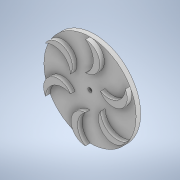
# Autodesk Inventor part: 20220608_ファン40mm羽数6枚
Saved by Autodesk Inventor 2020 (Build 240168000, 168)
## iProperties
Created: 2022-06-08
Part Number: 20220608_ファン40mm羽数6枚
Material: 一般
Document SubType Name: Modeling
Designer: Naggy
Density: 1 g/cm^3
Appearance: 既定
Author: Naggy
Autodesk Inventor part; units mm, degrees
ref_plane "YZ Plane" through (0, 0, 0) normal (1, 0, 0) x (0, 1, 0)
ref_plane "XZ Plane" through (0, 0, 0) normal (0, 1, 0) x (-1, 0, 0)
ref_plane "XY Plane" through (0, 0, 0) normal (0, 0, 1) x (1, 0, 0)
sketch "スケッチ1" plane through (0, 0, 0) normal (0, 0, 1) x (1, 0, 0)
  circle A0 centre (0, 0) radius 20
  dimension "d0" = 40
  constraints: 1 centre point, 1 coincident
  measures "d0" diameter of A0
extrude "押し出し1" add sketch "スケッチ1" along normal blind 2
sketch "スケッチ2" plane through (0, 0, 2) normal (0, 0, 1) x (1, 0, 0)
  circle A0 centre (0, 0) radius 7.5
  circle A1 centre (0, 0) radius 20 projected
  arc A2 (0, 7.5) -> (0, 20) centre (0, 13.75) ccw
  arc A3 (0, 7.5) -> (0, 20) centre (-4, 13.75) ccw
  arc A4 (-6.4952, 3.75) -> (-17.3205, 10) centre (-11.9078, 6.875) ccw
  arc A5 (-6.4952, 3.75) -> (-17.3205, 10) centre (-13.9078, 3.4109) ccw
  arc A6 (-6.4952, -3.75) -> (-17.3205, -10) centre (-11.9078, -6.875) ccw
  arc A7 (-6.4952, -3.75) -> (-17.3205, -10) centre (-9.9078, -10.3391) ccw
  arc A8 (0, -7.5) -> (0, -20) centre (0, -13.75) ccw
  arc A9 (0, -7.5) -> (0, -20) centre (4, -13.75) ccw
  arc A10 (6.4952, -3.75) -> (17.3205, -10) centre (11.9078, -6.875) ccw
  arc A11 (6.4952, -3.75) -> (17.3205, -10) centre (13.9078, -3.4109) ccw
  arc A12 (6.4952, 3.75) -> (17.3205, 10) centre (11.9078, 6.875) ccw
  arc A13 (6.4952, 3.75) -> (17.3205, 10) centre (9.9078, 10.3391) ccw
  dimension "d3" = 15
  dimension "d4" = 4
  dimension "d7" = 360
  constraints: 24 point on circle, 12 centre point, 2 vertical alignment, 1 coincident, 41 other
  measures "d4" distance of A3.centre A2.centre
extrude "押し出し2" add sketch "スケッチ2" along normal blind 2 contours A13 A12 | A11 A10 | A3 A2 | A9 A8 | A5 A4 | A7 A6
sketch "スケッチ3" plane through (0, 0, 2) normal (0, 0, 1) x (1, 0, 0)
  point P0 (0, 0)
  point P1 (0, 0)
  constraints: 1 coincident
hole "穴1" at (0, 0, 2) direction (0, 0, -1) diameter 1.8 depth 8.8 tip angle 118
